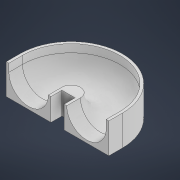
# Autodesk Inventor part: Troca de sentido
Saved by Autodesk Inventor 2022 (Build 260153000, 153)
## iProperties
Created: 2023-05-09
Part Number: Troca de sentido
Material: Genérico
Document SubType Name: Modeling
Designer: jpjoa
Density: 1 g/cm^3
Appearance: Padrão
Author: jpjoa
Autodesk Inventor part; units mm, degrees
ref_plane "YZ Plane" through (0, 0, 0) normal (1, 0, 0) x (0, 1, 0)
ref_plane "XZ Plane" through (0, 0, 0) normal (0, 1, 0) x (-1, 0, 0)
ref_plane "XY Plane" through (0, 0, 0) normal (0, 0, 1) x (1, 0, 0)
sketch "Esboço1" plane through (0, 0, 0) normal (0, 1, 0) x (-1, 0, 0)
  line L0 (-1.2, -1.2) -> (-19.2, -1.2)
  line L1 (-19.2, -1.2) -> (-19.2, -6.2)
  line L2 (-19.2, -6.2) -> (-27.6, -6.2)
  line L3 (-27.6, -6.2) -> (-27.6, -1.2)
  line L4 (-27.6, -1.2) -> (-45.6, -1.2)
  line L5 (-45.6, -1.2) -> (-45.6, -6.2)
  arc A0 (-45.6, -6.2) -> (-1.2, -6.2) centre (-23.4, -6.2) ccw
  line L6 (-23.4, -6.2) -> (-45.6, -6.2) construction
  line L7 (-23.4, -6.2) -> (-1.2, -6.2) construction
  line L8 (-1.2, -6.2) -> (-1.2, -1.2)
  arc A1 (-46.8, -6.2) -> (0, -6.2) centre (-23.4, -6.2) ccw
  line L9 (0, -6.2) -> (0, 0)
  line L10 (0, 0) -> (-20.4, 0)
  line L11 (-20.4, 0) -> (-20.4, -5)
  line L12 (-20.4, -5) -> (-26.4, -5)
  line L13 (-26.4, -5) -> (-26.4, 0)
  line L14 (-26.4, 0) -> (-46.8, 0)
  line L15 (-46.8, 0) -> (-46.8, -6.2)
  line L16 (-45.6, -1.2) -> (-45.6, 0)
  line L17 (-27.6, -1.2) -> (-27.6, 0)
  line L18 (-19.2, -1.2) -> (-19.2, 0)
  line L19 (-1.2, -1.2) -> (-1.2, 0)
  arc A2 (-27.6, -6.2) -> (-19.2, -6.2) centre (-23.4, -6.2) ccw
  point P0 (-46.8, -6.2)
  dimension "d0" = 18
  dimension "d1" = 180
  dimension "d3" = 1.2
  dimension "d4" = 6
  dimension "d5" = 5
  dimension "d7" = 18
  constraints: 40 end point, 11 perpendicular, 9 coincident, 7 point on line, 6 point on circle, 3 centre point, 2 horizontal alignment, 1 collinear, 1 horizontal, 1 midpoint, 1 vertical, 7 other
  measures "d0" distance of L0.start L0.end
  measures "d1" angle of L7 L6
  measures "d3" radial gap between concentric circles of A0 A1
  measures "d4" distance between parallel lines of L13 L11
  measures "d5" distance between parallel lines of L14 L12
  measures "d7" radial gap between concentric circles of A0 A2
extrude "Extrusão1" add sketch "Esboço1" against normal blind 1.2
extrude "Extrusão2" add sketch "Esboço1" along normal blind 9 contours L1 L2 L3 L17 L14 L13 L12 L11 L10 L18 | A2 L2
extrude "Extrusão3" add sketch "Esboço1" along normal blind 12.6 contours L19 L10 L9 A1 L15 L14 L16 L5 A0 L8
fillet "Arredondamento1" radius 9 6 edges at (1.2, 0, -3.1) (45.6, 0, -3.1) (23.4, 0, -28.4) (23.4, 0, -10.4) (19.2, 0, -3.1) (27.6, 0, -3.1)
equation "\"d0\" = Diâmetro_esfera"
equation "\"d3\" = Margem"
equation "\"d4\" = Espessura_torre_base"
equation "\"d8\" = Margem"
equation "\"d10\" = 0.5 * Diâmetro_esfera"
equation "\"d12\" = 0.7 * Diâmetro_esfera"
equation "\"d14\" = 0.5 * Diâmetro_esfera"
equation "\"Diâmetro_esfera\" = 18"
equation "\"Filamento\" = 0.4"
equation "\"Margem\" = 3 * Filamento"
equation "\"Espessura_torre_base\" = 15 * Filamento"
